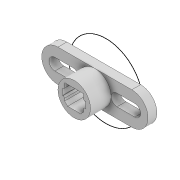
# Autodesk Inventor part: 00_toslink_launcher_largeholes_v3
Saved by Autodesk Inventor 2022 (Build 260153000, 153)
## iProperties
Created: 2022-08-14
Part Number: 00_toslink_launcher_largeholes_v3
Material: Generic
Document SubType Name: Modeling
Designer: diederichbenedict
Density: 1 g/cm^3
Appearance: Default
Author: diederichbenedict
Autodesk Inventor part; units mm, degrees
ref_plane "YZ Plane" through (0, 0, 0) normal (1, 0, 0) x (0, 1, 0)
ref_plane "XZ Plane" through (0, 0, 0) normal (0, 1, 0) x (-1, 0, 0)
ref_plane "XY Plane" through (0, 0, 0) normal (0, 0, 1) x (1, 0, 0)
sketch "Skizze1" plane through (-7.0778, 1.2599, 0) normal (0, 0, -1) x (-1, 0, 0)
  circle A0 centre (1.4222, -1.2599) radius 1.9 projected
  circle A1 centre (-7.0778, -1.2599) radius 3 projected
  circle A2 centre (-7.0778, -1.2599) radius 12.456
  point P0 (-7.0778, -1.2599)
  constraints: 1 centre point, 1 coincident
sketch "Skizze2" plane through (5.0781, 0.7351, 10.7) normal (0, 0, 1) x (1, 0, 0)
  line L0 (-8.9952, 0.4649) -> (-8.9952, -1.5851) projected
  circle A0 centre (-8.8322, -2.0851) radius 0.5 projected
  line L1 (-8.3322, -1.9739) -> (-8.3322, -2.9351) projected
  line L2 (-7.2781, -3.9351) -> (-8.3322, -2.9351) projected
  line L3 (-2.8781, -3.9351) -> (-7.2781, -3.9351) projected
  line L4 (-1.8781, -2.9351) -> (-2.8781, -3.9351) projected
  line L5 (-1.8781, -1.9239) -> (-1.8781, -2.9351) projected
  circle A1 centre (-1.3781, -2.0351) radius 0.5 projected
  line L6 (-1.1952, 0.4649) -> (-1.1952, -1.5351) projected
  line L7 (-1.4893, 0.4649) -> (-1.1952, 0.4649) projected
  line L8 (-1.1952, -1.5351) -> (-1.4893, -1.5351) projected
  circle A2 centre (-1.3781, 0.9649) radius 0.5 projected
  line L9 (-1.8781, 2.4649) -> (-1.8781, 0.8536) projected
  line L10 (-8.2781, 2.4649) -> (-1.8781, 2.4649) projected
  line L11 (-8.2781, 0.8536) -> (-8.2781, 2.4649) projected
  circle A3 centre (-8.7781, 0.9649) radius 0.5 projected
  line L12 (-8.9952, 0.4649) -> (-8.6668, 0.4649) projected
  line L13 (-8.721, -1.5851) -> (-8.9952, -1.5851) projected
  circle A4 centre (-5.0781, -0.7351) radius 5.5
  point P0 (-8.7794, 0.4649)
  point P1 (-8.2781, 0.9644)
  point P2 (-1.8781, 0.9649)
  point P3 (-1.3781, 0.4649)
  point P4 (-1.3774, -1.5351)
  point P5 (-1.8781, -2.0363)
  point P6 (-8.3322, -2.0847)
  point P7 (-8.8321, -1.5851)
  dimension "d0" = 11
  constraints: 1 centre point, 1 coincident
  measures "d0" diameter of A4
extrude "Extrusion1" add sketch "Skizze2" against normal blind 10 contours A3 | A0 | A2 | A1 | A4
sketch "Skizze3" plane through (0, 0, 0.7) normal (0, 0, -1) x (-1, 0, 0)
  circle A0 centre (0, 0) radius 5.5 projected
  line L0 (3.2542, -2.2) -> (2.2, -3.2) projected
  line L1 (2.2, -3.2) -> (-2.2, -3.2) projected
  line L2 (-2.2, -3.2) -> (-3.2, -2.2) projected
  line L3 (-3.2, -2.2) -> (-3.2, -1.3012) projected
  arc A1 (-3.2, -1.3012) -> (-3.7007, -0.8) centre (-3.7, -1.3) ccw projected
  line L4 (-3.7007, -0.8) -> (-3.8829, -0.8) projected
  line L5 (-3.8829, -0.8) -> (-3.8829, 1.2) projected
  line L6 (-3.8829, 1.2) -> (-3.7, 1.2) projected
  arc A2 (-3.7, 1.2) -> (-3.2, 1.7) centre (-3.7, 1.7) ccw projected
  line L7 (-3.2, 1.7) -> (-3.2, 3.2) projected
  line L8 (-3.2, 3.2) -> (3.2, 3.2) projected
  line L9 (3.2, 3.2) -> (3.2, 1.6995) projected
  arc A3 (3.2, 1.6995) -> (3.7013, 1.2) centre (3.7, 1.7) ccw projected
  line L10 (3.7013, 1.2) -> (3.9171, 1.2) projected
  line L11 (3.9171, 1.2) -> (3.9171, -0.85) projected
  line L12 (3.9171, -0.85) -> (3.7541, -0.85) projected
  arc A4 (3.7541, -0.85) -> (3.2542, -1.3496) centre (3.7542, -1.35) ccw projected
  line L13 (3.2542, -1.3496) -> (3.2542, -2.2) projected
  line L14 (-12.5, 0) -> (12.5, 0) construction
  line L15 (-12.5, -5.5) -> (12.5, -5.5)
  line L16 (12.5, 5.5) -> (-12.5, 5.5)
  arc A5 (-12.5, 5.5) -> (-12.5, -5.5) centre (-12.5, 0) ccw
  arc A6 (12.5, -5.5) -> (12.5, 5.5) centre (12.5, 0) ccw
  line L17 (13.5, 0) -> (7.5, 0) construction
  line L18 (13.5, 2) -> (7.5, 2)
  line L19 (7.5, -2) -> (13.5, -2)
  arc A7 (13.5, -2) -> (13.5, 2) centre (13.5, 0) ccw
  arc A8 (7.5, 2) -> (7.5, -2) centre (7.5, 0) ccw
  line L20 (-13.5, 0) -> (-7.5, 0) construction
  line L21 (-13.5, -2) -> (-7.5, -2)
  line L22 (-7.5, 2) -> (-13.5, 2)
  arc A9 (-13.5, 2) -> (-13.5, -2) centre (-13.5, 0) ccw
  arc A10 (-7.5, -2) -> (-7.5, 2) centre (-7.5, 0) ccw
  point P0 (0, 0)
  point P1 (10.5, 0)
  point P2 (-10.5, 0)
  point P3 (0, 5.5)
  point P4 (0, -5.5)
  dimension "d3" = 12.5
  dimension "d4" = 3
  dimension "d5" = 4
  dimension "d6" = 3
  dimension "d7" = 4
  dimension "d8" = 10.5
  dimension "d9" = 10.5
  constraints: 24 end point, 12 point on circle, 12 tangent, 6 centre point, 4 point on line, 3 midpoint, 3 parallel, 1 horizontal
  measures "d3" distance of point (0, 0) L14.end
  measures "d4" distance of point (10.5, 0) L17.end
  measures "d5" diameter of A8
  measures "d6" distance of point (-10.5, 0) L20.end
  measures "d7" diameter of A10
  measures "d8" distance of point (10.5, 0) point (0, 0)
  measures "d9" distance of point (0, 0) point (-10.5, 0)
extrude "Extrusion2" add sketch "Skizze3" against normal blind 3 contours A0 L16 A6 L15 | A0 L15 A5 L16
